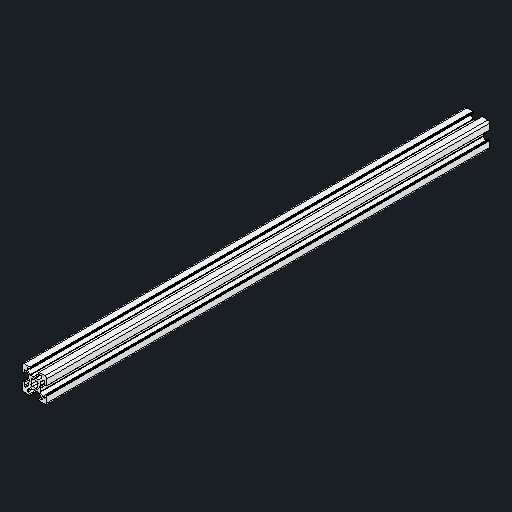
# Autodesk Inventor part: Al-profile-20x20-360
Saved by Autodesk Inventor 2026 (Build 300175050, 175E)
## iProperties
Created: 2020-02-13
Part Number: Al-profile-20x20-360
Material: Aluminum 6061
Document SubType Name: Modeling
Designer: kuzmin
Density: 2.7 g/cm^3
Appearance: Aluminum - Flat
Length: 360,000 mm
Author: kuzmin
Autodesk Inventor part; units mm, degrees
ref_plane "YZ Plane" through (0, 0, 0) normal (1, 0, 0) x (0, 1, 0)
ref_plane "XZ Plane" through (0, 0, 0) normal (0, 1, 0) x (-1, 0, 0)
ref_plane "XY Plane" through (0, 0, 0) normal (0, 0, 1) x (1, 0, 0)
sketch "Sketch2" plane through (0, 0, 0) normal (0, 0, 1) x (1, 0, 0)
  arc A0 (0.2, 0) -> (0, 0.2) centre (0, 0) ccw projected
  line L0 (0, 0.2) -> (-4.75, 0.2) projected
  arc A1 (-4.75, 0.2) -> (-6.25, -1.3) centre (-4.75, -1.3) ccw projected
  line L1 (-6.25, -1.3) -> (-6.25, -6.05) projected
  arc A2 (-6.25, -6.05) -> (-6.05, -6.25) centre (-6.05, -6.05) ccw projected
  line L2 (-6.05, -6.25) -> (-5.95, -6.25) projected
  arc A3 (-5.75, -6.45) -> (-5.95, -6.25) centre (-5.95, -6.45) ccw projected
  line L3 (-5.75, -6.45) -> (-5.75, -6.6) projected
  arc A4 (-5.75, -6.6) -> (-5.55, -6.8) centre (-5.55, -6.6) ccw projected
  line L4 (-5.55, -6.8) -> (-5.25, -6.8) projected
  arc A5 (-5.25, -6.8) -> (-4.75, -6.3) centre (-5.25, -6.3) ccw projected
  line L5 (-4.75, -6.3) -> (-4.75, -4.3) projected
  arc A6 (-4.25, -3.8) -> (-4.75, -4.3) centre (-4.25, -4.3) ccw projected
  line L6 (-4.25, -3.8) -> (-3.5178, -3.8) projected
  arc A7 (-3.1642, -3.9464) -> (-3.5178, -3.8) centre (-3.5178, -4.3) ccw projected
  line L7 (-3.1642, -3.9464) -> (-0.8964, -6.2142) projected
  arc A8 (-0.75, -6.5678) -> (-0.8964, -6.2142) centre (-1.25, -6.5678) ccw projected
  line L8 (-0.75, -6.5678) -> (-0.75, -8.8464) projected
  arc A9 (-0.75, -8.8464) -> (-0.7232, -8.9464) centre (-0.55, -8.8464) ccw projected
  line L9 (-0.7232, -8.9464) -> (-0.2881, -9.7) projected
  arc A10 (-0.2881, -9.9) -> (-0.2881, -9.7) centre (-0.4613, -9.8) ccw projected
  line L10 (-0.2881, -9.9) -> (-0.7232, -10.6536) projected
  arc A11 (-0.7232, -10.6536) -> (-0.75, -10.7536) centre (-0.55, -10.7536) ccw projected
  line L11 (-0.75, -10.7536) -> (-0.75, -13.0322) projected
  arc A12 (-0.8964, -13.3858) -> (-0.75, -13.0322) centre (-1.25, -13.0322) ccw projected
  line L12 (-0.8964, -13.3858) -> (-3.1642, -15.6536) projected
  arc A13 (-3.5178, -15.8) -> (-3.1642, -15.6536) centre (-3.5178, -15.3) ccw projected
  line L13 (-3.5178, -15.8) -> (-4.25, -15.8) projected
  arc A14 (-4.75, -15.3) -> (-4.25, -15.8) centre (-4.25, -15.3) ccw projected
  line L14 (-4.75, -15.3) -> (-4.75, -13.3) projected
  arc A15 (-4.75, -13.3) -> (-5.25, -12.8) centre (-5.25, -13.3) ccw projected
  line L15 (-5.25, -12.8) -> (-5.55, -12.8) projected
  arc A16 (-5.55, -12.8) -> (-5.75, -13) centre (-5.55, -13) ccw projected
  line L16 (-5.75, -13) -> (-5.75, -13.15) projected
  arc A17 (-5.95, -13.35) -> (-5.75, -13.15) centre (-5.95, -13.15) ccw projected
  line L17 (-5.95, -13.35) -> (-6.05, -13.35) projected
  arc A18 (-6.05, -13.35) -> (-6.25, -13.55) centre (-6.05, -13.55) ccw projected
  line L18 (-6.25, -13.55) -> (-6.25, -18.3) projected
  arc A19 (-6.25, -18.3) -> (-4.75, -19.8) centre (-4.75, -18.3) ccw projected
  line L19 (-4.75, -19.8) -> (0, -19.8) projected
  arc A20 (0, -19.8) -> (0.2, -19.6) centre (0, -19.6) ccw projected
  line L20 (0.2, -19.6) -> (0.2, -19.5) projected
  arc A21 (0.4, -19.3) -> (0.2, -19.5) centre (0.4, -19.5) ccw projected
  line L21 (0.4, -19.3) -> (0.55, -19.3) projected
  arc A22 (0.55, -19.3) -> (0.75, -19.1) centre (0.55, -19.1) ccw projected
  line L22 (0.75, -19.1) -> (0.75, -18.8) projected
  arc A23 (0.75, -18.8) -> (0.25, -18.3) centre (0.25, -18.8) ccw projected
  line L23 (0.25, -18.3) -> (-1.75, -18.3) projected
  arc A24 (-2.25, -17.8) -> (-1.75, -18.3) centre (-1.75, -17.8) ccw projected
  line L24 (-2.25, -17.8) -> (-2.25, -17.0678) projected
  arc A25 (-2.1036, -16.7142) -> (-2.25, -17.0678) centre (-1.75, -17.0678) ccw projected
  line L25 (-2.1036, -16.7142) -> (0.1642, -14.4464) projected
  arc A26 (0.5178, -14.3) -> (0.1642, -14.4464) centre (0.5178, -14.8) ccw projected
  line L26 (0.5178, -14.3) -> (2.7964, -14.3) projected
  arc A27 (2.7964, -14.3) -> (2.8964, -14.2732) centre (2.7964, -14.1) ccw projected
  line L27 (2.8964, -14.2732) -> (3.65, -13.8381) projected
  arc A28 (3.85, -13.8381) -> (3.65, -13.8381) centre (3.75, -14.0113) ccw projected
  line L28 (3.85, -13.8381) -> (4.6036, -14.2732) projected
  arc A29 (4.6036, -14.2732) -> (4.7036, -14.3) centre (4.7036, -14.1) ccw projected
  line L29 (4.7036, -14.3) -> (6.9822, -14.3) projected
  arc A30 (7.3358, -14.4464) -> (6.9822, -14.3) centre (6.9822, -14.8) ccw projected
  line L30 (7.3358, -14.4464) -> (9.6036, -16.7142) projected
  arc A31 (9.75, -17.0678) -> (9.6036, -16.7142) centre (9.25, -17.0678) ccw projected
  line L31 (9.75, -17.0678) -> (9.75, -17.8) projected
  arc A32 (9.25, -18.3) -> (9.75, -17.8) centre (9.25, -17.8) ccw projected
  line L32 (9.25, -18.3) -> (7.25, -18.3) projected
  arc A33 (7.25, -18.3) -> (6.75, -18.8) centre (7.25, -18.8) ccw projected
  line L33 (6.75, -18.8) -> (6.75, -19.1) projected
  arc A34 (6.75, -19.1) -> (6.95, -19.3) centre (6.95, -19.1) ccw projected
  line L34 (6.95, -19.3) -> (7.1, -19.3) projected
  arc A35 (7.3, -19.5) -> (7.1, -19.3) centre (7.1, -19.5) ccw projected
  line L35 (7.3, -19.5) -> (7.3, -19.6) projected
  arc A36 (7.3, -19.6) -> (7.5, -19.8) centre (7.5, -19.6) ccw projected
  line L36 (7.5, -19.8) -> (12.25, -19.8) projected
  arc A37 (12.25, -19.8) -> (13.75, -18.3) centre (12.25, -18.3) ccw projected
  line L37 (13.75, -18.3) -> (13.75, -13.55) projected
  arc A38 (13.75, -13.55) -> (13.55, -13.35) centre (13.55, -13.55) ccw projected
  line L38 (13.55, -13.35) -> (13.45, -13.35) projected
  arc A39 (13.25, -13.15) -> (13.45, -13.35) centre (13.45, -13.15) ccw projected
  line L39 (13.25, -13.15) -> (13.25, -13) projected
  arc A40 (13.25, -13) -> (13.05, -12.8) centre (13.05, -13) ccw projected
  line L40 (13.05, -12.8) -> (12.75, -12.8) projected
  arc A41 (12.75, -12.8) -> (12.25, -13.3) centre (12.75, -13.3) ccw projected
  line L41 (12.25, -13.3) -> (12.25, -15.3) projected
  arc A42 (11.75, -15.8) -> (12.25, -15.3) centre (11.75, -15.3) ccw projected
  line L42 (11.75, -15.8) -> (11.0178, -15.8) projected
  arc A43 (10.6642, -15.6536) -> (11.0178, -15.8) centre (11.0178, -15.3) ccw projected
  line L43 (10.6642, -15.6536) -> (8.3964, -13.3858) projected
  arc A44 (8.25, -13.0322) -> (8.3964, -13.3858) centre (8.75, -13.0322) ccw projected
  line L44 (8.25, -13.0322) -> (8.25, -10.7536) projected
  arc A45 (8.25, -10.7536) -> (8.2232, -10.6536) centre (8.05, -10.7536) ccw projected
  line L45 (8.2232, -10.6536) -> (7.7881, -9.9) projected
  arc A46 (7.7881, -9.7) -> (7.7881, -9.9) centre (7.9613, -9.8) ccw projected
  line L46 (7.7881, -9.7) -> (8.2232, -8.9464) projected
  arc A47 (8.2232, -8.9464) -> (8.25, -8.8464) centre (8.05, -8.8464) ccw projected
  line L47 (8.25, -8.8464) -> (8.25, -6.5678) projected
  arc A48 (8.3964, -6.2142) -> (8.25, -6.5678) centre (8.75, -6.5678) ccw projected
  line L48 (8.3964, -6.2142) -> (10.6642, -3.9464) projected
  arc A49 (11.0178, -3.8) -> (10.6642, -3.9464) centre (11.0178, -4.3) ccw projected
  line L49 (11.0178, -3.8) -> (11.75, -3.8) projected
  arc A50 (12.25, -4.3) -> (11.75, -3.8) centre (11.75, -4.3) ccw projected
  line L50 (12.25, -4.3) -> (12.25, -6.3) projected
  arc A51 (12.25, -6.3) -> (12.75, -6.8) centre (12.75, -6.3) ccw projected
  line L51 (12.75, -6.8) -> (13.05, -6.8) projected
  arc A52 (13.05, -6.8) -> (13.25, -6.6) centre (13.05, -6.6) ccw projected
  line L52 (13.25, -6.6) -> (13.25, -6.45) projected
  arc A53 (13.45, -6.25) -> (13.25, -6.45) centre (13.45, -6.45) ccw projected
  line L53 (13.45, -6.25) -> (13.55, -6.25) projected
  arc A54 (13.55, -6.25) -> (13.75, -6.05) centre (13.55, -6.05) ccw projected
  line L54 (13.75, -6.05) -> (13.75, -1.3) projected
  arc A55 (13.75, -1.3) -> (12.25, 0.2) centre (12.25, -1.3) ccw projected
  line L55 (12.25, 0.2) -> (7.5, 0.2) projected
  arc A56 (7.5, 0.2) -> (7.3, 0) centre (7.5, 0) ccw projected
  line L56 (7.3, 0) -> (7.3, -0.1) projected
  arc A57 (7.1, -0.3) -> (7.3, -0.1) centre (7.1, -0.1) ccw projected
  line L57 (7.1, -0.3) -> (6.95, -0.3) projected
  arc A58 (6.95, -0.3) -> (6.75, -0.5) centre (6.95, -0.5) ccw projected
  line L58 (6.75, -0.5) -> (6.75, -0.8) projected
  arc A59 (6.75, -0.8) -> (7.25, -1.3) centre (7.25, -0.8) ccw projected
  line L59 (7.25, -1.3) -> (9.25, -1.3) projected
  arc A60 (9.75, -1.8) -> (9.25, -1.3) centre (9.25, -1.8) ccw projected
  line L60 (9.75, -1.8) -> (9.75, -2.5322) projected
  arc A61 (9.6036, -2.8858) -> (9.75, -2.5322) centre (9.25, -2.5322) ccw projected
  line L61 (9.6036, -2.8858) -> (7.3358, -5.1536) projected
  arc A62 (6.9822, -5.3) -> (7.3358, -5.1536) centre (6.9822, -4.8) ccw projected
  line L62 (6.9822, -5.3) -> (4.7036, -5.3) projected
  arc A63 (4.7036, -5.3) -> (4.6036, -5.3268) centre (4.7036, -5.5) ccw projected
  line L63 (4.6036, -5.3268) -> (3.85, -5.7619) projected
  arc A64 (3.65, -5.7619) -> (3.85, -5.7619) centre (3.75, -5.5887) ccw projected
  line L64 (3.65, -5.7619) -> (2.8964, -5.3268) projected
  arc A65 (2.8964, -5.3268) -> (2.7964, -5.3) centre (2.7964, -5.5) ccw projected
  line L65 (2.7964, -5.3) -> (0.5178, -5.3) projected
  arc A66 (0.1642, -5.1536) -> (0.5178, -5.3) centre (0.5178, -4.8) ccw projected
  line L66 (0.1642, -5.1536) -> (-2.1036, -2.8858) projected
  arc A67 (-2.25, -2.5322) -> (-2.1036, -2.8858) centre (-1.75, -2.5322) ccw projected
  line L67 (-2.25, -2.5322) -> (-2.25, -1.8) projected
  arc A68 (-1.75, -1.3) -> (-2.25, -1.8) centre (-1.75, -1.8) ccw projected
  line L68 (-1.75, -1.3) -> (0.25, -1.3) projected
  arc A69 (0.25, -1.3) -> (0.75, -0.8) centre (0.25, -0.8) ccw projected
  line L69 (0.75, -0.8) -> (0.75, -0.5) projected
  arc A70 (0.75, -0.5) -> (0.55, -0.3) centre (0.55, -0.5) ccw projected
  line L70 (0.55, -0.3) -> (0.4, -0.3) projected
  arc A71 (0.2, -0.1) -> (0.4, -0.3) centre (0.4, -0.1) ccw projected
  line L71 (0.2, -0.1) -> (0.2, 0) projected
  line L72 (1.3047, -11.0582) -> (0.7578, -11.7099) projected
  arc A72 (1.3047, -8.5418) -> (1.3047, -11.0582) centre (3.75, -9.8) ccw projected
  line L73 (0.7578, -7.8901) -> (1.3047, -8.5418) projected
  arc A73 (1.8361, -6.8104) -> (0.7578, -7.8901) centre (3.75, -9.8) ccw projected
  line L74 (2.4918, -7.3547) -> (1.8361, -6.8104) projected
  arc A74 (5.0082, -7.3547) -> (2.4918, -7.3547) centre (3.75, -9.8) ccw projected
  line L75 (5.6639, -6.8104) -> (5.0082, -7.3547) projected
  arc A75 (6.7422, -7.8901) -> (5.6639, -6.8104) centre (3.75, -9.8) ccw projected
  line L76 (6.1953, -8.5418) -> (6.7422, -7.8901) projected
  arc A76 (6.1953, -11.0582) -> (6.1953, -8.5418) centre (3.75, -9.8) ccw projected
  line L77 (6.7422, -11.7099) -> (6.1953, -11.0582) projected
  arc A77 (5.6639, -12.7896) -> (6.7422, -11.7099) centre (3.75, -9.8) ccw projected
  line L78 (5.0082, -12.2453) -> (5.6639, -12.7896) projected
  arc A78 (2.4918, -12.2453) -> (5.0082, -12.2453) centre (3.75, -9.8) ccw projected
  line L79 (1.8361, -12.7896) -> (2.4918, -12.2453) projected
  arc A79 (0.7578, -11.7099) -> (1.8361, -12.7896) centre (3.75, -9.8) ccw projected
extrude "Extrusion2" add sketch "Sketch2" along normal mid plane 360
equation "\"d2\" = Length"
equation "\"Length\" = 360"
body "Solid2"
